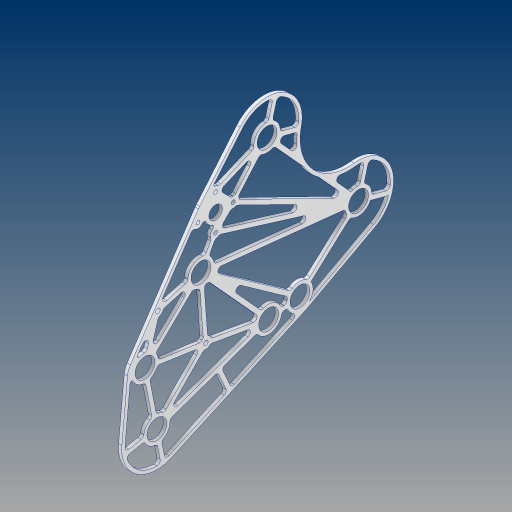
# Autodesk Inventor part: SHOT_1_001_ShooterPlate
Saved by Autodesk Inventor 2024.3 (Build 283343000, 343)
## iProperties
Created: 2024-08-07
Part Number: SHOT_1_001_ShooterPlate
Material: Aluminum 6061
Document SubType Name: Modeling
Designer: Kenji
Density: 2.7 g/cm^3
Appearance: Aluminum - Flat
Mass: 320.131 g
Surface Area: 825.953 cm^2
Volume: 118.567 cm^3
Author: Kenji
Autodesk Inventor part; units mm, degrees
ref_plane "YZ Plane" through (0, 0, 0) normal (1, 0, 0) x (0, 1, 0)
ref_plane "XZ Plane" through (0, 0, 0) normal (0, 1, 0) x (-1, 0, 0)
ref_plane "XY Plane" through (0, 0, 0) normal (0, 0, 1) x (1, 0, 0)
sketch "Sketch1" plane through (0, 0, 0) normal (1, 0, 0) x (0, 1, 0)
  line L0 (0, 0) -> (355.6, 0) construction
  line L1 (0, -355.6) -> (0, 0) construction
  line L2 (0, -292.1) -> (279.4, -292.1) construction
  circle A0 centre (336.7111, -261.0807) radius 50.8 construction
  circle A1 centre (191.0749, -393.5194) radius 50.8 construction
  circle A2 centre (263.893, -327.3) radius 50.8 construction
  circle A3 centre (191.0749, -393.5194) radius 47.625 construction
  circle A4 centre (336.7111, -261.0807) radius 47.625 construction
  line L3 (336.7111, -261.0807) -> (191.0749, -393.5194) construction
  circle A5 centre (336.7111, -261.0807) radius 14.2875
  circle A6 centre (191.0749, -393.5194) radius 14.2875
  circle A7 centre (215.3861, -165.4189) radius 25.4 construction
  circle A8 centre (107.6199, -263.4195) radius 25.4 construction
  circle A9 centre (107.6199, -263.4195) radius 22.225 construction
  circle A10 centre (215.3861, -165.4189) radius 22.225 construction
  circle A11 centre (215.3861, -165.4189) radius 14.2875
  circle A12 centre (107.6199, -263.4195) radius 14.2875
  line L4 (301.4765, -293.1223) -> (198.9433, -180.3717) construction
  line L5 (226.3095, -361.4778) -> (123.7762, -248.7272) construction
  circle A13 centre (161.3597, -214.5495) radius 50.8 construction
  line L6 (215.3861, -165.4189) -> (107.6199, -263.4195) construction
  circle A14 centre (50.8, -101.6) radius 50.8 construction
  circle A15 centre (25.4, -170.0653) radius 25.4 construction
  circle A16 centre (25.4, -170.0653) radius 22.225 construction
  circle A17 centre (25.4, -170.0653) radius 14.2875 construction
  circle A18 centre (136.3874, -84.4507) radius 25.4 construction
  circle A19 centre (136.3874, -84.4507) radius 22.225 construction
  circle A20 centre (136.3874, -84.4507) radius 14.2875
  circle A21 centre (50.8, -101.6) radius 14.2875
  circle A22 centre (41.2055, -25.7462) radius 25.4 construction
  circle A23 centre (41.2055, -25.7462) radius 22.225 construction
  circle A24 centre (41.2055, -25.7462) radius 14.2875 construction
  circle A25 centre (-111.1945, -98.7712) radius 50.8 construction
  circle A26 centre (41.2055, -98.7712) radius 50.8 construction
  line L7 (-111.1945, -47.9712) -> (41.2055, -47.9712) construction
  line L8 (-111.1945, -149.5712) -> (41.2055, -149.5712) construction
  circle A27 centre (280.082, -186.6804) radius 30 construction
  circle A28 centre (280.082, -186.6804) radius 25.4 construction
  circle A29 centre (305.482, -186.6804) radius 2.794
  circle A30 centre (298.0425, -168.7199) radius 2.794
  circle A31 centre (280.082, -161.2804) radius 2.794
  circle A32 centre (262.1215, -168.7199) radius 2.794
  circle A33 centre (254.682, -186.6804) radius 2.794
  circle A34 centre (262.1215, -204.6409) radius 2.794
  circle A35 centre (280.082, -212.0804) radius 2.794
  circle A36 centre (298.0425, -204.6409) radius 2.794
  circle A37 centre (280.082, -186.6804) radius 9.652
  line L9 (298.2517, -210.5522) -> (305.9436, -220.6579) construction
  line L10 (251.5816, -177.3141) -> (239.5164, -173.3491) construction
  circle A38 centre (280.082, -186.6804) radius 9.5504 construction
  circle A39 centre (336.7111, -261.0807) radius 9.5504 construction
  line L11 (344.3106, -255.2964) -> (287.6815, -180.8961) construction
  line L12 (329.1116, -266.8649) -> (272.4825, -192.4647) construction
  circle A40 centre (336.7111, -261.0807) radius 14.3256 construction
  circle A41 centre (215.3861, -165.4189) radius 14.3256 construction
  line L13 (206.5162, -176.6683) -> (327.8412, -272.33) construction
  line L14 (224.2559, -154.1696) -> (345.5809, -249.8313) construction
  circle A42 centre (136.3874, -84.4507) radius 14.3256 construction
  circle A43 centre (215.3861, -165.4189) radius 14.3256 construction
  line L15 (225.6397, -155.4147) -> (146.6411, -74.4464) construction
  line L16 (205.1324, -175.4232) -> (126.1337, -94.4549) construction
  circle A44 centre (107.6199, -263.4195) radius 22.86 construction
  circle A45 centre (113.7181, -308.7309) radius 22.86 construction
  circle A46 centre (113.7181, -308.7309) radius 14.2875
  circle A47 centre (113.7181, -308.7309) radius 9.5504 construction
  line L17 (119.3674, -316.4313) -> (285.7312, -194.3808) construction
  line L18 (274.4327, -178.98) -> (108.0688, -301.0306) construction
  circle A48 centre (123.5241, -172.549) radius 6.35 construction
  circle A49 centre (123.5241, -172.549) radius 3.2512
  line L19 (122.4294, -178.8039) -> (111.9989, -238.3998) construction
  arc A50 (325.875, -310.7115) -> (241.5089, -387.4324) centre (310.9541, -379.0508) ccw
  line L20 (146.341, -417.5925) -> (93.5878, -319.5638)
  line L21 (369.2764, -222.0917) -> (299.3135, -163.6555)
  line L22 (296.8294, -161.7902) -> (150.5669, -63.377)
  arc A51 (325.875, -310.7115) -> (369.2764, -222.0917) centre (336.7111, -261.0807) ccw
  arc A52 (146.341, -417.5925) -> (241.5089, -387.4324) centre (191.0749, -393.5194) ccw
  arc A53 (92.8854, -318.1427) -> (93.5878, -319.5638) centre (113.7181, -308.7309) ccw
  arc A54 (299.3135, -163.6555) -> (296.8294, -161.7902) centre (280.082, -186.6804) ccw
  line L23 (138.8602, -59.1713) -> (55.7455, -51.0413)
  line L24 (92.8854, -318.1427) -> (4.5052, -122.5149)
  arc A55 (150.5669, -63.377) -> (138.8602, -59.1713) centre (136.3874, -84.4507) ccw
  arc A56 (55.7455, -51.0413) -> (4.5052, -122.5149) centre (50.8, -101.6) ccw
  circle A57 centre (198.2507, -103.1148) radius 6.35 construction
  circle A58 centre (198.2507, -103.1148) radius 3.2512
  line L25 (193.7057, -107.5493) -> (186.1404, -114.9306) construction
  line L26 (161.503, -214.4192) -> (263.893, -327.3) construction
  point P0 (33.8339, -53.7169)
  dimension "d38" = 50.8
  dimension "d44" = 101.6
  dimension "d82" = 50.8
  dimension "d102" = 12.7
  dimension "d108" = 12.7
  dimension "d13" = 355.6
  dimension "d14" = 355.6
  dimension "d15" = 292.1
  dimension "d29" = 101.6
  dimension "d31" = 3.175
  dimension "d36" = 28.575
  dimension "d39" = 3.175
  dimension "d41" = 28.575
  dimension "d42" = 152.4
  dimension "d43" = 152.4
  dimension "d46" = 279.4
  dimension "d47" = 101.6
  dimension "d50" = 101.6
  dimension "d51" = 145.6628
  dimension "d60" = 28.575
  dimension "d61" = 113.1223
  dimension "d77" = 101.6
  dimension "d78" = 101.6
  dimension "d79" = 152.4
  dimension "d80" = 41.2055
  dimension "d81" = 60
  dimension "d83" = 5.588
  dimension "d86" = 360
  dimension "d88" = 19.304
  dimension "d90" = 12.7
  dimension "d91" = 19.1008
  dimension "d92" = 19.1008
  dimension "d93" = 28.6512
  dimension "d94" = 28.6512
  dimension "d95" = 28.6512
  dimension "d96" = 28.6512
  dimension "d97" = 45.72
  dimension "d99" = 28.575
  dimension "d100" = 19.1008
  dimension "d101" = 206.3329
  dimension "d103" = 6.5024
  dimension "d109" = 6.5024
  dimension "d111" = 56.5611
  dimension "d114" = 101.6
  dimension "d116" = 87.2886
  dimension "d117" = 158.0611
  dimension "d119" = 323.8734
  dimension "d121" = 42.21
  constraints: 54 end point, 52 centre point, 52 point on circle, 43 tangent, 23 coincident, 14 equal radius, 10 point on line, 5 concentric, 4 midpoint, 3 horizontal, 2 horizontal alignment, 2 perpendicular, 1 equal length, 1 parallel, 1 vertical alignment, 45 other
  measures "d13" distance of L1.start L0.start
  measures "d14" distance of L0.start L0.end
  measures "d15" distance between parallel lines of L0 L2
  measures "d29" diameter of A1
  measures "d31" radial gap between concentric circles of A1 A3
  measures "d36" diameter of A5
  measures "d41" diameter of A12
  measures "d42" distance of L4.start L4.end
  measures "d43" distance of L5.start L5.end
  measures "d46" distance of L2.start L2.end
  measures "d47" diameter of A14
  measures "d50" distance from line of L0 A14.centre
  measures "d51" distance of L6.start L6.end
  measures "d60" diameter of A21
  measures "d61" distance of A19.centre point (215.386, -165.419)
  measures "d77" diameter of A25
  measures "d78" diameter of A26
  measures "d79" distance of L8.start L8.end
  measures "d80" distance from line of L1 A22.centre
  measures "d81" diameter of A27
  measures "d83" diameter of A29
  measures "d88" diameter of A37
  measures "d90" distance of L9.start L9.end
  measures "d91" diameter of A38
  measures "d92" diameter of A39
  measures "d93" diameter of A40
  measures "d94" diameter of A41
  measures "d95" diameter of A42
  measures "d96" diameter of A43
  measures "d97" diameter of A44
  measures "d99" diameter of A46
  measures "d100" diameter of A47
  measures "d101" distance of L17.start L17.end
  measures "d103" diameter of A49
  measures "d109" diameter of A58
  measures "d111" distance of L15.end L25.end
  measures "d114" distance of point (123.524, -172.549) A14.centre
  measures "d116" distance of A14.centre A19.centre
  measures "d117" distance of A14.centre L26.start
  measures "d119" distance of A14.centre L3.end
  measures "d121" angle of L1 L26
extrude "Extrusion2" add sketch "Sketch1" along normal blind 4.7625 contours A30 | A32 | A34 | A36 | A50 A52 L20 A53 L24 A56 L23 A55 L22 A54 L21 A51
sketch "Sketch2" plane through (4.7625, 0, 0) normal (1, 0, 0) x (0, 0, -1)
  line L0 (59.1713, 138.8602) -> (51.0413, 55.7455) projected
  arc A0 (51.0413, 55.7455) -> (122.5149, 4.5052) centre (101.6, 50.8) ccw projected
  line L1 (122.5149, 4.5052) -> (318.1427, 92.8854) projected
  arc A1 (318.1427, 92.8854) -> (319.5638, 93.5878) centre (308.7309, 113.7181) ccw projected
  line L2 (319.5638, 93.5878) -> (417.5925, 146.341) projected
  arc A2 (417.5925, 146.341) -> (387.4324, 241.5089) centre (393.5194, 191.0749) ccw projected
  arc A3 (310.7115, 325.875) -> (387.4324, 241.5089) centre (379.0508, 310.9541) ccw projected
  arc A4 (310.7115, 325.875) -> (222.0917, 369.2764) centre (261.0807, 336.7111) ccw projected
  line L3 (222.0917, 369.2764) -> (163.6555, 299.3135) projected
  arc A5 (163.6555, 299.3135) -> (161.7902, 296.8294) centre (186.6804, 280.082) ccw projected
  line L4 (161.7902, 296.8294) -> (63.377, 150.5669) projected
  arc A6 (63.377, 150.5669) -> (59.1713, 138.8602) centre (84.4507, 136.3874) ccw projected
  circle A7 centre (308.7309, 113.7181) radius 14.2875 projected
  circle A8 centre (212.0804, 280.082) radius 2.794 projected
  circle A9 centre (186.6804, 254.682) radius 2.794 projected
  circle A10 centre (161.2804, 280.082) radius 2.794 projected
  circle A11 centre (186.6804, 305.482) radius 2.794 projected
  circle A12 centre (165.4189, 215.3861) radius 14.2875 projected
  circle A13 centre (103.1148, 198.2507) radius 3.2512 projected
  circle A14 centre (172.549, 123.5241) radius 3.2512 projected
  circle A15 centre (186.6804, 280.082) radius 9.652 projected
  circle A16 centre (101.6, 50.8) radius 14.2875 projected
  circle A17 centre (84.4507, 136.3874) radius 14.2875 projected
  circle A18 centre (263.4195, 107.6199) radius 14.2875 projected
  circle A19 centre (393.5194, 191.0749) radius 14.2875 projected
  circle A20 centre (261.0807, 336.7111) radius 14.2875 projected
  arc A21 (306.0462, 326.8936) -> (225.7567, 366.2153) centre (261.0807, 336.7111) ccw construction
  arc A22 (306.0462, 326.8936) -> (388.0046, 236.7681) centre (379.0508, 310.9541) ccw construction
  arc A23 (415.3297, 150.546) -> (388.0046, 236.7681) centre (393.5194, 191.0749) ccw construction
  line L5 (415.3297, 150.546) -> (317.301, 97.7928) construction
  arc A24 (316.1767, 97.2371) -> (317.301, 97.7928) centre (308.7309, 113.7181) ccw construction
  line L6 (316.1767, 97.2371) -> (120.5489, 8.8569) construction
  arc A25 (55.7938, 55.2806) -> (120.5489, 8.8569) centre (101.6, 50.8) ccw construction
  line L7 (55.7938, 55.2806) -> (64.0193, 139.3706) construction
  line L8 (73.6429, 157.2702) -> (165.7521, 294.1637) construction
  arc A26 (167.3204, 296.2523) -> (165.7521, 294.1637) centre (186.6804, 280.082) ccw construction
  line L9 (167.3204, 296.2523) -> (225.7567, 366.2153) construction
  circle A27 centre (261.0807, 336.7111) radius 19.0627 construction
  circle A28 centre (212.0804, 280.082) radius 7.5692 construction
  circle A29 centre (186.6804, 305.482) radius 7.5692 construction
  circle A30 centre (161.2804, 280.082) radius 7.5692 construction
  circle A31 centre (186.6804, 280.082) radius 14.4272 construction
  circle A32 centre (186.6804, 254.682) radius 7.5692 construction
  circle A33 centre (165.4189, 215.3861) radius 19.0627 construction
  circle A34 centre (393.5194, 191.0749) radius 19.0627 construction
  circle A35 centre (103.1148, 198.2507) radius 8.0264 construction
  circle A36 centre (84.4507, 136.3874) radius 19.0627 construction
  circle A37 centre (172.549, 123.5241) radius 8.0264 construction
  circle A38 centre (263.4195, 107.6199) radius 19.0627 construction
  circle A39 centre (308.7309, 113.7181) radius 19.0627 construction
  circle A40 centre (101.6, 50.8) radius 19.0627 construction
  line L10 (379.437, 178.2268) -> (322.8133, 126.5662) construction
  line L11 (374.5641, 193.0952) -> (184.3743, 213.3658) construction
  line L12 (166.8941, 196.3805) -> (171.9279, 131.5264) construction
  line L13 (244.6422, 110.9063) -> (180.4552, 122.1404) construction
  line L14 (250.5943, 121.7231) -> (178.2441, 201.2828) construction
  line L15 (293.1833, 124.7479) -> (180.9666, 204.3563) construction
  line L16 (370.8364, 190.2995) -> (195.3573, 209.0022)
  line L17 (292.2388, 129.3107) -> (192.0882, 200.3592)
  line L18 (374.7777, 178.2738) -> (323.1928, 131.2102)
  line L19 (282.3118, 110.1625) -> (289.8386, 111.1755) construction
  arc A41 (195.3573, 209.0022) -> (192.0882, 200.3592) centre (194.8512, 204.2539) ccw
  arc A42 (374.9756, 186.6577) -> (375.9583, 183.6591) centre (393.5194, 191.0749) ccw
  arc A43 (317.7221, 130.5272) -> (297.752, 129.3017) centre (308.7309, 113.7181) ccw
  arc A44 (292.2388, 129.3107) -> (297.752, 129.3017) centre (295.0018, 133.2054) ccw
  arc A45 (317.7221, 130.5272) -> (323.1928, 131.2102) centre (319.9744, 134.7379) ccw
  arc A46 (374.7777, 178.2738) -> (375.9583, 183.6591) centre (371.5593, 181.8014) ccw
  arc A47 (374.9756, 186.6577) -> (370.8364, 190.2995) centre (370.3303, 185.5512) ccw
  line L20 (288.5646, 124.1316) -> (223.4422, 170.3305)
  line L21 (250.6487, 126.3824) -> (217.1464, 163.2232)
  line L22 (285.2683, 113.764) -> (286.0352, 113.8672)
  arc A48 (223.4422, 170.3305) -> (217.1464, 163.2232) centre (220.6793, 166.4359) ccw
  arc A49 (280.3822, 116.3177) -> (256.0321, 125.193) centre (263.4195, 107.6199) ccw
  arc A50 (290.3949, 118.9311) -> (290.0722, 117.6219) centre (308.7309, 113.7181) ccw
  arc A51 (250.6487, 126.3824) -> (256.0321, 125.193) centre (254.1816, 129.5951) ccw
  arc A52 (280.3822, 116.3177) -> (285.2683, 113.764) centre (284.6313, 118.4966) ccw
  arc A53 (286.0352, 113.8672) -> (290.0722, 117.6219) centre (285.3982, 118.5998) ccw
  arc A54 (290.3949, 118.9311) -> (288.5646, 124.1316) centre (285.8017, 120.2369) ccw
  line L23 (245.4433, 122.6682) -> (178.6728, 196.0923)
  line L24 (170.3791, 192.5101) -> (174.938, 133.7734)
  line L25 (241.0872, 114.7518) -> (182.9799, 124.9218)
  arc A55 (179.6052, 127.3496) -> (177.0319, 130.182) centre (172.549, 123.5241) ccw
  arc A56 (248.4244, 119.39) -> (245.4518, 113.9879) centre (263.4195, 107.6199) ccw construction
  arc A57 (170.039, 196.8917) -> (175.716, 199.3437) centre (165.4189, 215.3861) ccw construction
  arc A58 (178.6728, 196.0923) -> (170.3791, 192.5101) centre (175.1399, 192.8796) ccw
  arc A59 (174.938, 133.7734) -> (177.0319, 130.182) centre (179.6989, 134.143) ccw
  arc A60 (179.6052, 127.3496) -> (182.9799, 124.9218) centre (183.8031, 129.6255) ccw
  arc A61 (241.0872, 114.7518) -> (245.4433, 122.6682) centre (241.9105, 119.4555) ccw
  line L26 (245.4333, 101.3044) -> (119.5861, 57.1155) construction
  line L27 (97.8548, 69.4912) -> (88.1959, 117.6962) construction
  line L28 (164.6068, 124.6838) -> (103.3134, 133.6332) construction
  line L29 (166.944, 117.7789) -> (114.9118, 64.4449) construction
  line L30 (232.8884, 109.7402) -> (181.8851, 118.6668)
  line L31 (167.8149, 114.1249) -> (127.5798, 72.8832)
  line L32 (233.6472, 100.531) -> (132.5799, 65.0431)
  arc A62 (244.3571, 107.733) -> (244.6327, 104.3883) centre (263.4195, 107.6199) ccw
  arc A63 (171.7239, 115.5402) -> (177.8864, 117.5295) centre (172.549, 123.5241) ccw
  arc A64 (118.283, 60.023) -> (116.9985, 62.0371) centre (101.6, 50.8) ccw construction
  arc A65 (127.5798, 72.8832) -> (132.5799, 65.0431) centre (130.9979, 69.5486) ccw
  arc A66 (171.7239, 115.5402) -> (167.8149, 114.1249) centre (171.233, 110.7903) ccw
  arc A67 (181.8851, 118.6668) -> (177.8864, 117.5295) centre (181.0619, 113.9631) ccw
  arc A68 (233.6472, 100.531) -> (232.8884, 109.7402) centre (232.0652, 105.0365) ccw
  line L33 (105.3452, 32.1088) -> (110.6423, 5.6722) construction
  line L34 (82.9088, 47.0548) -> (56.4722, 41.7577) construction
  line L35 (185.2344, 76.8016) -> (123.8558, 55.2497)
  line L36 (109.1283, 29.3887) -> (112.5581, 12.2719)
  line L37 (286.1152, 107.4708) -> (286.8821, 107.574)
  arc A69 (111.3645, 34.428) -> (120.6626, 50.7553) centre (101.6, 50.8) ccw
  arc A70 (248.5694, 95.6674) -> (282.0781, 103.7161) centre (263.4195, 107.6199) ccw
  arc A71 (291.7682, 105.0202) -> (298.671, 97.526) centre (308.7309, 113.7181) ccw
  line L38 (199.1805, 44.735) -> (119.1947, 8.8532)
  arc A72 (123.8558, 55.2497) -> (120.6626, 50.7553) centre (125.4378, 50.7442) ccw
  arc A73 (111.3645, 34.428) -> (109.1283, 29.3887) centre (113.8105, 30.3268) ccw
  arc A74 (112.5581, 12.2719) -> (119.1947, 8.8532) centre (117.2402, 13.2101) ccw
  arc A75 (248.5694, 95.6674) -> (243.2674, 97.1789) centre (244.8494, 92.6733) ccw
  arc A76 (286.1152, 107.4708) -> (282.0781, 103.7161) centre (286.7521, 102.7382) ccw
  arc A77 (291.7682, 105.0202) -> (286.8821, 107.574) centre (287.5191, 102.8414) ccw
  arc A78 (298.1055, 89.113) -> (298.671, 97.526) centre (296.151, 93.4698) ccw
  line L39 (398.4532, 209.4881) -> (405.4315, 235.5315) construction
  line L40 (411.9326, 186.1411) -> (437.976, 179.1628) construction
  line L41 (393.5194, 191.0749) -> (412.5821, 191.0749) construction
  line L42 (379.0576, 173.5828) -> (324.7565, 124.0412)
  line L43 (410.8536, 183.1432) -> (437.0483, 176.1244)
  arc A79 (384.5283, 174.2658) -> (410.8536, 183.1432) centre (393.5194, 191.0749) ccw
  arc A80 (322.6084, 100.6489) -> (324.7565, 124.0412) centre (308.7309, 113.7181) ccw
  line L44 (322.6084, 100.6489) -> (415.3297, 150.546)
  arc A81 (415.3297, 150.546) -> (437.0483, 176.1244) centre (393.5194, 191.0749) ccw
  arc A82 (384.5283, 174.2658) -> (379.0576, 173.5828) centre (382.276, 170.0551) ccw
  line L45 (402.4027, 211.9605) -> (407.0623, 229.3502)
  line L46 (416.0485, 188.3253) -> (433.4382, 183.6657)
  arc A83 (412.5238, 192.5646) -> (404.3117, 206.7884) centre (393.5194, 191.0749) ccw
  arc A84 (439.4383, 187.9544) -> (413.7765, 232.4021) centre (393.5194, 191.0749) ccw
  arc A85 (413.7765, 232.4021) -> (407.0623, 229.3502) centre (411.6747, 228.1143) ccw
  arc A86 (433.4382, 183.6657) -> (439.4383, 187.9544) centre (434.6741, 188.2782) ccw
  arc A87 (412.5238, 192.5646) -> (416.0485, 188.3253) centre (417.2844, 192.9377) ccw
  arc A88 (402.4027, 211.9605) -> (404.3117, 206.7884) centre (407.0152, 210.7246) ccw
  line L47 (147.0387, 210.331) -> (110.8539, 200.3792) construction
  line L48 (100.7965, 190.5664) -> (89.9568, 154.6376) construction
  line L49 (98.095, 149.6998) -> (151.7747, 202.0737) construction
  line L50 (102.7533, 149.8089) -> (151.5509, 197.4195)
  line L51 (163.9925, 192.7347) -> (168.6071, 133.282)
  line L52 (163.0793, 128.1155) -> (107.1467, 136.2822)
  arc A89 (167.0925, 129.4105) -> (167.0442, 129.3654) centre (172.549, 123.5241) ccw
  arc A90 (103.152, 140.0818) -> (101.7536, 144.3871) centre (84.4507, 136.3874) ccw
  arc A91 (156.9957, 198.2853) -> (160.4711, 196.9767) centre (165.4189, 215.3861) ccw
  arc A92 (102.7533, 149.8089) -> (101.7536, 144.3871) centre (106.088, 146.391) ccw
  arc A93 (103.152, 140.0818) -> (107.1467, 136.2822) centre (107.8366, 141.0073) ccw
  arc A94 (163.0793, 128.1155) -> (167.0442, 129.3654) centre (163.7692, 132.8406) ccw
  arc A95 (167.0925, 129.4105) -> (168.6071, 133.282) centre (163.8462, 132.9125) ccw
  arc A96 (156.9957, 198.2853) -> (151.5509, 197.4195) centre (154.8856, 194.0016) ccw
  arc A97 (163.9925, 192.7347) -> (160.4711, 196.9767) centre (159.2317, 192.3651) ccw
  line L53 (156.6558, 122.636) -> (106.2293, 129.9988)
  line L54 (100.2979, 73.4589) -> (91.979, 114.9761)
  line L55 (159.384, 114.5763) -> (115.0207, 69.1031)
  arc A98 (164.7959, 121.4475) -> (165.1286, 120.4647) centre (172.549, 123.5241) ccw construction
  arc A99 (94.2152, 120.0154) -> (101.3149, 127.5) centre (84.4507, 136.3874) ccw
  arc A100 (109.5989, 68.1033) -> (104.303, 69.6701) centre (101.6, 50.8) ccw
  arc A101 (159.384, 114.5763) -> (156.6558, 122.636) centre (155.9659, 117.9109) ccw
  arc A102 (106.2293, 129.9988) -> (101.3149, 127.5) centre (105.5394, 125.2737) ccw
  arc A103 (94.2152, 120.0154) -> (91.979, 114.9761) centre (96.6612, 115.9142) ccw
  arc A104 (100.2979, 73.4589) -> (104.303, 69.6701) centre (104.98, 74.3971) ccw
  arc A105 (109.5989, 68.1033) -> (115.0207, 69.1031) centre (111.6027, 72.4377) ccw
  line L56 (80.1887, 43.2717) -> (62.5364, 39.7347)
  line L57 (102.9021, 28.1411) -> (106.4391, 10.4889)
  arc A106 (59.0611, 33.2295) -> (101.7751, 4.7755) centre (101.6, 50.8) ccw
  arc A107 (85.228, 41.0355) -> (98.897, 31.9299) centre (101.6, 50.8) ccw
  arc A108 (85.228, 41.0355) -> (80.1887, 43.2717) centre (81.1268, 38.5895) ccw
  arc A109 (102.9021, 28.1411) -> (98.897, 31.9299) centre (98.22, 27.2029) ccw
  arc A110 (101.7751, 4.7755) -> (106.4391, 10.4889) centre (101.757, 9.5507) ccw
  arc A111 (62.5364, 39.7347) -> (59.0611, 33.2295) centre (63.4746, 35.0525) ccw
  line L58 (65.588, 139.1416) -> (64.0193, 139.3706) construction
  line L59 (78.9411, 49.4979) -> (61.2889, 45.9609)
  line L60 (94.0717, 72.2113) -> (85.7528, 113.7285)
  arc A112 (67.3435, 127.9774) -> (81.7477, 117.5173) centre (84.4507, 136.3874) ccw
  line L61 (62.8245, 127.1564) -> (55.7938, 55.2806)
  arc A113 (55.7938, 55.2806) -> (55.5755, 50.6249) centre (101.6, 50.8) ccw
  arc A114 (55.5755, 50.6249) -> (61.2889, 45.9609) centre (60.3507, 50.643) ccw
  arc A115 (91.8355, 67.172) -> (82.7299, 53.503) centre (101.6, 50.8) ccw
  arc A116 (78.9411, 49.4979) -> (82.7299, 53.503) centre (78.0029, 54.18) ccw
  arc A117 (91.8355, 67.172) -> (94.0717, 72.2113) centre (89.3895, 71.2732) ccw
  arc A118 (85.7528, 113.7285) -> (81.7477, 117.5173) centre (81.0707, 112.7903) ccw
  circle A119 centre (65.2008, 126.924) radius 2.3876 construction
  arc A120 (67.3435, 127.9774) -> (62.8245, 127.1564) centre (65.2008, 126.924) ccw
  line L62 (89.4966, 164.1046) -> (87.9022, 158.8197)
  arc A121 (83.5549, 155.429) -> (76.6063, 153.7613) centre (84.4507, 136.3874) ccw
  arc A122 (97.4146, 192.6) -> (97.9459, 192.1103) centre (103.1148, 198.2507) ccw construction
  line L63 (73.6429, 157.2702) -> (80.9631, 168.1496)
  arc A123 (89.4966, 164.1046) -> (80.9631, 168.1496) centre (84.9249, 165.4839) ccw
  arc A124 (83.5549, 155.429) -> (87.9022, 158.8197) centre (83.3305, 160.199) ccw
  circle A125 centre (75.6238, 155.9374) radius 2.3876 construction
  arc A126 (73.6429, 157.2702) -> (76.6063, 153.7613) centre (75.6238, 155.9374) ccw
  line L64 (136.5314, 204.1483) -> (113.6313, 197.8502)
  line L65 (103.2564, 187.7276) -> (96.3963, 164.9895)
  line L66 (104.3027, 160.1923) -> (141.1324, 196.1262)
  arc A127 (106.0699, 190.7881) -> (110.5024, 195.1128) centre (103.1148, 198.2507) ccw
  arc A128 (148.1374, 207.3403) -> (149.748, 204.5322) centre (165.4189, 215.3861) ccw construction
  arc A129 (95.6872, 151.7864) -> (92.9195, 153.4656) centre (84.4507, 136.3874) ccw construction
  arc A130 (113.6313, 197.8502) -> (110.5024, 195.1128) centre (114.8976, 193.2459) ccw
  arc A131 (106.0699, 190.7881) -> (103.2564, 187.7276) centre (107.828, 186.3484) ccw
  arc A132 (141.1324, 196.1262) -> (136.5314, 204.1483) centre (137.7977, 199.5441) ccw
  arc A133 (96.3963, 164.9895) -> (104.3027, 160.1923) centre (100.968, 163.6102) ccw
  line L67 (186.6804, 265.6548) -> (186.6804, 262.2512) construction
  line L68 (168.8496, 280.082) -> (172.2532, 280.082) construction
  line L69 (183.0785, 248.0247) -> (174.4903, 232.152) construction
  line L70 (169.5385, 276.907) -> (170.8124, 276.907)
  line L71 (183.5054, 264.2139) -> (183.5054, 264.1254)
  line L72 (179.3941, 247.8872) -> (173.3208, 236.6624)
  line L73 (142.9085, 212.488) -> (115.9222, 205.066)
  line L74 (110.694, 212.336) -> (150.9539, 272.1706)
  arc A134 (157.3778, 273.5964) -> (167.5582, 275.8533) centre (161.2804, 280.082) ccw
  arc A135 (173.0655, 275.3092) -> (181.9077, 266.4671) centre (186.6804, 280.082) ccw
  arc A136 (181.8056, 260.4724) -> (179.6375, 251.909) centre (186.6804, 254.682) ccw
  arc A137 (168.3793, 234.2175) -> (146.4051, 216.7504) centre (165.4189, 215.3861) ccw
  arc A138 (157.3778, 273.5964) -> (150.9539, 272.1706) centre (154.9158, 269.5048) ccw
  arc A139 (179.3941, 247.8872) -> (179.6375, 251.909) centre (175.1942, 250.1596) ccw
  arc A140 (168.3793, 234.2175) -> (173.3208, 236.6624) centre (169.1209, 238.9348) ccw
  arc A141 (142.9085, 212.488) -> (146.4051, 216.7504) centre (141.6422, 217.0922) ccw
  arc A142 (110.694, 212.336) -> (115.9222, 205.066) centre (114.6559, 209.6702) ccw
  circle A143 centre (181.1178, 264.2139) radius 2.3876 construction
  circle A144 centre (170.8124, 274.5194) radius 2.3876 construction
  circle A145 centre (169.5385, 274.5194) radius 2.3876 construction
  arc A146 (169.5385, 276.907) -> (167.5582, 275.8533) centre (169.5385, 274.5194) ccw
  arc A147 (173.0655, 275.3092) -> (170.8124, 276.907) centre (170.8124, 274.5194) ccw
  arc A148 (181.8056, 260.4724) -> (183.5054, 264.1254) centre (178.7302, 264.1254) ccw
  arc A149 (183.5054, 264.2139) -> (181.9077, 266.4671) centre (181.1178, 264.2139) ccw
  line L75 (193.9153, 252.4571) -> (375.2988, 196.6781) construction
  line L76 (204.5112, 280.082) -> (201.1076, 280.082) construction
  line L77 (181.3282, 300.1297) -> (166.6327, 285.4342) construction
  line L78 (192.0327, 300.1297) -> (206.7282, 285.4342) construction
  line L79 (186.6804, 297.9128) -> (186.6804, 294.5092) construction
  line L80 (217.0332, 285.8058) -> (248.6073, 322.2957) construction
  line L81 (193.6597, 308.4115) -> (243.5036, 329.3332) construction
  line L82 (206.7282, 274.7297) -> (192.0327, 260.0342) construction
  line L83 (218.876, 276.7483) -> (376.4051, 199.4705) construction
  line L84 (184.979, 244.8654) -> (178.9057, 233.6406)
  line L85 (194.7735, 248.8715) -> (313.7398, 212.287)
  line L86 (311.8301, 202.9744) -> (188.102, 216.1615)
  arc A150 (188.2124, 247.2694) -> (190.7822, 248.3205) centre (186.6804, 254.682) ccw
  arc A151 (183.9628, 219.8033) -> (179.5626, 228.1667) centre (165.4189, 215.3861) ccw
  arc A152 (194.7735, 248.8715) -> (190.7822, 248.3205) centre (193.3699, 244.3072) ccw
  arc A153 (188.2124, 247.2694) -> (184.979, 244.8654) centre (189.1789, 242.593) ccw
  arc A154 (178.9057, 233.6406) -> (179.5626, 228.1667) centre (183.1056, 231.3682) ccw
  arc A155 (183.9628, 219.8033) -> (188.102, 216.1615) centre (188.608, 220.9098) ccw
  arc A156 (311.8301, 202.9744) -> (313.7398, 212.287) centre (312.3362, 207.7227) ccw
  line L87 (207.648, 271.1594) -> (198.2642, 261.7756)
  line L88 (200.2371, 253.8347) -> (298.2964, 223.6796)
  line L89 (219.1603, 273.0724) -> (301.8031, 232.531)
  arc A157 (211.433, 272.5405) -> (215.132, 273.1552) centre (212.0804, 280.082) ccw
  arc A158 (194.1813, 255.6971) -> (193.7841, 257.2955) centre (186.6804, 254.682) ccw construction
  arc A159 (198.2642, 261.7756) -> (200.2371, 253.8347) centre (201.6407, 258.399) ccw
  arc A160 (211.433, 272.5405) -> (207.648, 271.1594) centre (211.0245, 267.7828) ccw
  arc A161 (219.1603, 273.0724) -> (215.132, 273.1552) centre (217.0572, 268.7853) ccw
  arc A162 (298.2964, 223.6796) -> (301.8031, 232.531) centre (299.7, 228.2439) ccw
  line L90 (266.0144, 355.1242) -> (272.9928, 381.1676) construction
  line L91 (279.4938, 331.7773) -> (305.5372, 324.799) construction
  line L92 (261.0807, 336.7111) -> (280.1434, 336.7111) construction
  line L93 (179.8174, 311.2143) -> (180.8711, 310.3342) construction
  line L94 (194.1591, 312.0644) -> (239.1302, 330.9408)
  line L95 (263.8303, 359.2402) -> (268.4899, 376.6298)
  line L96 (184.6221, 316.9668) -> (225.7567, 366.2153)
  arc A163 (264.2011, 382.63) -> (225.7567, 366.2153) centre (261.0807, 336.7111) ccw
  arc A164 (259.591, 355.7155) -> (242.0493, 335.6177) centre (261.0807, 336.7111) ccw
  arc A165 (190.1329, 312.2179) -> (186.5087, 313.0492) centre (186.6804, 305.482) ccw
  arc A166 (190.1329, 312.2179) -> (194.1591, 312.0644) centre (192.3109, 316.4675) ccw
  arc A167 (239.1302, 330.9408) -> (242.0493, 335.6177) centre (237.282, 335.3439) ccw
  arc A168 (259.591, 355.7155) -> (263.8303, 359.2402) centre (259.2178, 360.4761) ccw
  arc A169 (268.4899, 376.6298) -> (264.2011, 382.63) centre (263.8774, 377.8658) ccw
  circle A170 centre (186.4545, 315.4362) radius 2.3876 construction
  arc A171 (184.6221, 316.9668) -> (186.5087, 313.0492) centre (186.4545, 315.4362) ccw
  line L97 (198.8245, 307.136) -> (231.0073, 320.6446)
  line L98 (215.8586, 289.3007) -> (236.4665, 313.117)
  line L99 (197.2961, 299.3564) -> (207.648, 289.0045)
  arc A172 (212.1829, 287.6505) -> (211.433, 287.6234) centre (212.0804, 280.082) ccw
  arc A173 (193.7841, 302.8684) -> (194.2449, 305.2137) centre (186.6804, 305.482) ccw construction
  arc A174 (243.5036, 329.3332) -> (246.3806, 324.5746) centre (261.0807, 336.7111) ccw construction
  arc A175 (236.4665, 313.117) -> (231.0073, 320.6446) centre (232.8554, 316.2415) ccw
  arc A176 (212.1829, 287.6505) -> (215.8586, 289.3007) centre (212.2476, 292.4252) ccw
  arc A177 (207.648, 289.0045) -> (211.433, 287.6234) centre (211.0245, 292.3811) ccw
  arc A178 (198.8245, 307.136) -> (197.2961, 299.3564) centre (200.6727, 302.733) ccw
  line L100 (192.3828, 79.3117) -> (206.4342, 47.989) construction
  line L101 (191.1734, 74.2506) -> (201.5828, 51.0464)
  line L102 (197.5151, 75.6281) -> (207.4907, 53.391)
  arc A179 (191.1734, 74.2506) -> (185.2344, 76.8016) centre (186.8165, 72.2961) ccw
  arc A180 (199.1805, 44.735) -> (201.5828, 51.0464) centre (197.226, 49.0919) ccw
  line L103 (200.29, 82.0881) -> (243.2674, 97.1789)
  line L104 (213.8152, 50.9945) -> (298.1055, 89.113)
  arc A181 (200.29, 82.0881) -> (197.5151, 75.6281) centre (201.872, 77.5826) ccw
  arc A182 (207.4907, 53.391) -> (213.8152, 50.9945) centre (211.8476, 55.3455) ccw
  line L105 (273.9059, 322.6079) -> (380.6942, 205.1781) construction
  line L106 (273.8514, 317.9486) -> (314.2736, 273.4983)
  line L107 (335.6285, 250.0154) -> (363.1129, 219.7923)
  arc A183 (314.8439, 272.7284) -> (334.9161, 250.656) centre (379.0508, 310.9541) ccw
  line L108 (221.2289, 285.8025) -> (248.7767, 317.6393)
  line L109 (222.7368, 278.3908) -> (357.4769, 212.2924)
  arc A184 (357.4769, 212.2924) -> (363.1129, 219.7923) centre (359.58, 216.5796) ccw
  arc A185 (254.1291, 318.9611) -> (268.468, 319.138) centre (261.0807, 336.7111) ccw
  arc A186 (221.2289, 285.8025) -> (222.7368, 278.3908) centre (224.8399, 282.6779) ccw
  arc A187 (254.1291, 318.9611) -> (248.7767, 317.6393) centre (252.3878, 314.5147) ccw
  arc A188 (273.8514, 317.9486) -> (268.468, 319.138) centre (270.3185, 314.7359) ccw
  arc A189 (314.8439, 272.7284) -> (314.2736, 273.4983) centre (310.7408, 270.2856) ccw
  arc A190 (335.6285, 250.0154) -> (334.9161, 250.656) centre (332.0957, 246.8027) ccw
  line L110 (396.2691, 213.604) -> (400.9286, 230.9937)
  line L111 (363.1288, 229.2131) -> (380.7487, 209.8374)
  arc A191 (367.4058, 237.1427) -> (388.0046, 236.7681) centre (379.0508, 310.9541) ccw
  arc A192 (396.6399, 236.9938) -> (388.0046, 236.7681) centre (393.5194, 191.0749) ccw
  arc A193 (392.0298, 210.0793) -> (386.1321, 208.648) centre (393.5194, 191.0749) ccw
  arc A194 (367.4058, 237.1427) -> (363.1288, 229.2131) centre (366.6616, 232.4258) ccw
  arc A195 (400.9286, 230.9937) -> (396.6399, 236.9938) centre (396.3161, 232.2296) ccw
  arc A196 (392.0298, 210.0793) -> (396.2691, 213.604) centre (391.6566, 214.8399) ccw
  arc A197 (380.7487, 209.8374) -> (386.1321, 208.648) centre (384.2816, 213.0501) ccw
  line L112 (269.9639, 357.5967) -> (274.6235, 374.9863)
  line L113 (283.6097, 333.9614) -> (300.9994, 329.3019)
  line L114 (286.4207, 326.6342) -> (301.1077, 322.6989)
  line L115 (281.6519, 318.809) -> (296.1693, 302.8451)
  arc A198 (306.9996, 333.5906) -> (281.3377, 378.0382) centre (261.0807, 336.7111) ccw
  arc A199 (280.0851, 338.2008) -> (271.873, 352.4245) centre (261.0807, 336.7111) ccw
  arc A200 (304.6277, 317.658) -> (304.4682, 306.3519) centre (379.0508, 310.9541) ccw
  arc A201 (286.4207, 326.6342) -> (281.6519, 318.809) centre (285.1848, 322.0217) ccw
  arc A202 (304.6277, 317.658) -> (301.1077, 322.6989) centre (299.8718, 318.0864) ccw
  arc A203 (296.1693, 302.8451) -> (304.4682, 306.3519) centre (299.7021, 306.0578) ccw
  arc A204 (269.9639, 357.5967) -> (271.873, 352.4245) centre (274.5764, 356.3608) ccw
  arc A205 (280.0851, 338.2008) -> (283.6097, 333.9614) centre (284.8457, 338.5739) ccw
  arc A206 (300.9994, 329.3019) -> (306.9996, 333.5906) centre (302.2353, 333.9144) ccw
  arc A207 (281.3377, 378.0382) -> (274.6235, 374.9863) centre (279.236, 373.7504) ccw
  point P0 (0, 0)
  point P1 (374.4924, 189.9098)
  point P2 (183.773, 210.2369)
  point P3 (295.2375, 127.1834)
  point P4 (182.5865, 207.0999)
  point P5 (377.4938, 180.7518)
  point P6 (320.4767, 128.7322)
  point P7 (291.5634, 122.0043)
  point P8 (253.1224, 123.6622)
  point P9 (281.6245, 113.2736)
  point P10 (289.679, 114.3576)
  point P11 (291.5634, 122.0043)
  point P12 (175.144, 131.1194)
  point P13 (180.3578, 125.3807)
  point P14 (179.263, 119.1258)
  point P15 (169.6738, 116.0304)
  point P16 (246.7364, 98.3969)
  point P17 (120.3868, 54.0316)
  point P18 (108.406, 32.9937)
  point P19 (113.7339, 6.4035)
  point P20 (282.4714, 106.9804)
  point P21 (290.5259, 108.0644)
  point P22 (310.684, 94.7557)
  point P23 (381.7737, 176.0608)
  point P24 (401.4511, 208.4091)
  point P25 (408.47, 234.6038)
  point P26 (412.4971, 189.2768)
  point P27 (438.6918, 182.258)
  point P28 (100.1217, 147.2413)
  point P29 (154.1825, 199.9871)
  point P30 (163.708, 196.4003)
  point P31 (168.8131, 130.628)
  point P32 (165.7134, 127.7309)
  point P33 (103.5086, 136.8134)
  point P34 (102.5912, 130.53)
  point P35 (101.0202, 69.8539)
  point P36 (91.2567, 118.5811)
  point P37 (112.4532, 66.4714)
  point P38 (83.7937, 43.994)
  point P39 (57.2035, 38.6661)
  point P40 (102.1798, 31.7461)
  point P41 (107.5077, 5.1559)
  point P42 (82.5461, 50.2202)
  point P43 (55.9559, 44.8923)
  point P44 (94.794, 68.6063)
  point P45 (85.0304, 117.3335)
  point P46 (86.8402, 155.2997)
  point P47 (111.0646, 197.1443)
  point P48 (104.0252, 190.2761)
  point P49 (183.5054, 261.5531)
  point P50 (180.6182, 250.1496)
  point P51 (171.5712, 233.4287)
  point P52 (146.4535, 213.4629)
  point P53 (109.3807, 203.2669)
  point P54 (106.2019, 205.6597)
  point P55 (154.303, 277.148)
  point P56 (186.2031, 247.1278)
  point P57 (177.1561, 230.4069)
  point P58 (192.3148, 249.6276)
  point P59 (184.446, 216.5511)
  point P60 (209.4669, 272.9783)
  point P61 (216.8509, 274.2053)
  point P62 (191.7872, 311.0689)
  point P63 (242.5203, 332.3638)
  point P64 (262.8787, 355.6888)
  point P65 (269.8976, 381.8835)
  point P66 (244.9779, 326.5087)
  point P67 (214.1755, 287.3555)
  point P68 (209.4669, 287.1856)
  point P69 (195.3891, 80.3673)
  point P70 (209.4511, 49.021)
  point P71 (271.3777, 320.6687)
  point P72 (314.6026, 273.1366)
  point P73 (335.2995, 250.3772)
  point P74 (378.5244, 202.845)
  point P75 (218.9774, 283.2004)
  point P76 (251.1825, 320.4196)
  point P77 (219.6476, 279.9063)
  point P78 (378.0425, 202.2038)
  point P79 (395.3175, 210.0526)
  point P80 (402.3363, 236.2473)
  point P81 (352.2145, 241.215)
  point P82 (383.2223, 207.1172)
  point P83 (269.0123, 354.0453)
  point P84 (276.0312, 380.24)
  point P85 (280.0584, 334.913)
  point P86 (306.253, 327.8942)
  point P87 (278.4149, 328.7794)
  point P88 (305.0931, 321.631)
  point P89 (276.0757, 324.941)
  point P90 (307.0835, 290.8432)
  dimension "d122" = 4.7752
  dimension "d123" = 4.7752
  dimension "d124" = 4.7752
  dimension "d125" = 4.7752
  dimension "d126" = 4.7752
  dimension "d127" = 4.7752
  dimension "d128" = 4.7752
  dimension "d129" = 4.7752
  dimension "d130" = 4.7752
  dimension "d131" = 4.7752
  dimension "d132" = 4.7752
  dimension "d133" = 4.7752
  dimension "d134" = 4.7752
  dimension "d135" = 4.7752
  dimension "d136" = 4.7752
  dimension "d137" = 3.175
  dimension "d138" = 3.175
  dimension "d139" = 3.175
  dimension "d140" = 4.7752
  dimension "d141" = 4.7752
  dimension "d142" = 3.175
  dimension "d143" = 3.175
  dimension "d144" = 3.175
  dimension "d145" = 4.7752
  dimension "d146" = 4.7752
  dimension "d147" = 3.175
  dimension "d148" = 3.175
  dimension "d149" = 3.175
  dimension "d150" = 4.7752
  dimension "d151" = 3.175
  dimension "d152" = 3.175
  dimension "d153" = 3.175
  dimension "d154" = 4.7752
  dimension "d155" = 4.7752
  dimension "d156" = 90
  dimension "d157" = 3.175
  dimension "d158" = 3.175
  dimension "d159" = 3.175
  dimension "d160" = 4.7752
  dimension "d161" = 90
  dimension "d162" = 75
  dimension "d163" = 3.175
  dimension "d164" = 3.175
  dimension "d165" = 4.7752
  dimension "d166" = 3.175
  dimension "d167" = 3.175
  dimension "d168" = 4.7752
  dimension "d169" = 3.175
  dimension "d170" = 3.175
  dimension "d171" = 3.175
  dimension "d172" = 4.7752
  dimension "d173" = 4.7752
  dimension "d174" = 4.7752
  dimension "d175" = 3.175
  dimension "d176" = 3.175
  dimension "d177" = 3.175
  dimension "d178" = 4.7752
  dimension "d179" = 4.7752
  dimension "d180" = 3.175
  dimension "d181" = 3.175
  dimension "d182" = 4.7752
  dimension "d184" = 3.175
  dimension "d185" = 3.175
  dimension "d186" = 4.7752
  constraints: 452 point on circle, 222 end point, 216 tangent, 188 point on line, 175 centre point, 60 equal radius, 60 parallel, 16 concentric, 5 collinear, 3 horizontal, 2 perpendicular, 2 vertical, 238 other
  measures "d122" radial gap between concentric circles of A4 A21
  measures "d126" radial gap between concentric circles of A10 A30
  measures "d127" radial gap between concentric circles of A15 A31
  measures "d137" distance between parallel lines of L11 L16
  measures "d138" distance between parallel lines of L15 L17
  measures "d139" distance between parallel lines of L10 L18
  measures "d140" radius of A41
  measures "d141" radius of A44
  measures "d142" distance between parallel lines of L15 L20
  measures "d143" distance between parallel lines of L14 L21
  measures "d144" distance between parallel lines of L19 L22
  measures "d145" radius of A48
  measures "d146" radius of A51
  measures "d147" distance between parallel lines of L14 L23
  measures "d148" distance between parallel lines of L12 L24
  measures "d149" distance between parallel lines of L13 L25
  measures "d150" radius of A58
  measures "d151" distance between parallel lines of L13 L30
  measures "d152" distance between parallel lines of L29 L31
  measures "d153" distance between parallel lines of L26 L32
  measures "d154" radius of A65
  measures "d155" radius of A66
  measures "d156" angle of L33 L34
  measures "d157" distance between parallel lines of L26 L35
  measures "d158" distance between parallel lines of L33 L36
  measures "d159" distance between parallel lines of L19 L37
  measures "d160" radius of A72
  measures "d161" angle of L40 L39
  measures "d162" angle of L41 L39
  measures "d163" distance between parallel lines of L10 L42
  measures "d164" distance between parallel lines of L40 L43
  measures "d165" radius of A82
  measures "d166" distance between parallel lines of L39 L45
  measures "d167" distance between parallel lines of L40 L46
  measures "d168" radius of A85
  measures "d169" distance between parallel lines of L49 L50
  measures "d170" distance between parallel lines of L12 L51
  measures "d171" distance between parallel lines of L28 L52
  measures "d172" radius of A92
  measures "d173" radius of A94
  measures "d174" radius of A96
  measures "d175" distance between parallel lines of L28 L53
  measures "d176" distance between parallel lines of L27 L54
  measures "d177" distance between parallel lines of L29 L55
  measures "d178" radius of A101
  measures "d179" radius of A102
  measures "d180" distance between parallel lines of L34 L56
  measures "d181" distance between parallel lines of L33 L57
  measures "d182" radius of A108
  measures "d184" distance between parallel lines of L34 L59
  measures "d185" distance between parallel lines of L27 L60
  measures "d186" radius of A114
extrude "Extrusion3" cut sketch "Sketch2" against normal blind 25.4 contours A47 A42 A46 L18 A45 A43 A44 L17 A41 L16 | A54 A50 A53 L22 A52 A49 A51 L21 A48 L20 | A61 L25 A60 A55 A59 L24 A58 L23 | A68 L32 A65 L31 A66 A63 A67 L30 | A179 L101 A180 L38 A74 L36 A73 A69 A72 L35 | L37 A77 A71 A78 L104 A182 L102 A181 L103 A75 A70 A76 | A82 A79 L43 A81 L44 A80 L42 | L45 A85 A84 A86 L46 A87 A83 A88 | L50 A96 A91 A97 L51 A95 A89 A94 L52 A93 A90 A92 | A101 L55 A105 A100 A104 L54 A103 A99 A102 L53 | A108 A107 A109 L57 A110 A106 A111 L56 | L59 A114 A113 L61 A120 A112 A118 L60 A117 A115 A116 | L62 A124 A121 A126 L63 A123 | A132 L66 A133 L65 A131 A127 A130 L64 | L70 A147 A135 A149 L71 A148 A136 A139 L72 A140 A137 A141 L73 A142 L74 A138 A134 A146 | A153 A150 A152 L85 A156 L86 A155 A151 A154 L84 | A160 A157 A161 L89 A162 L88 A159 L87 | A166 A165 A171 L96 A163 A169 L95 A168 A164 A167 L94 | L97 A175 L98 A176 A172 A177 L99 A178 | L106 A189 A183 A190 L107 A184 L109 A186 L108 A187 A185 A188 | A196 A193 A197 L111 A194 A191 A192 A195 L110 | L112 A207 A198 A206 L113 A205 A199 A204 | L114 A202 A200 A203 L115 A201
body "Solid2"
